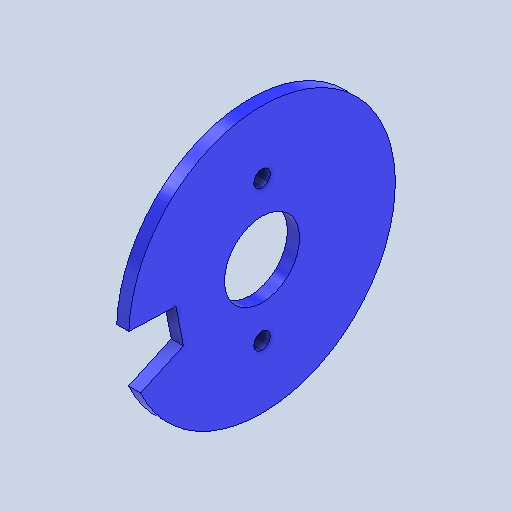
# Autodesk Inventor part: belt_liner_v2_3DP_P-2-F
Saved by Autodesk Inventor 2025.2 (Build 292293000, 293)
## iProperties
Created: 2025-01-13
Part Number: belt_liner_v2_3DP_P-2-F
Material: ABS プラスチック
Document SubType Name: Modeling
Designer: haruy
Density: 1.06 g/cm^3
Appearance: 青 - 壁塗料 - 光沢
Author: haruy
Autodesk Inventor part; units mm, degrees
ref_plane "YZ Plane" through (0, 0, 0) normal (1, 0, 0) x (0, 1, 0)
ref_plane "XZ Plane" through (0, 0, 0) normal (0, 1, 0) x (-1, 0, 0)
ref_plane "XY Plane" through (0, 0, 0) normal (0, 0, 1) x (1, 0, 0)
sketch "スケッチ1" plane through (0, 0, 0) normal (1, 0, 0) x (0, 1, 0)
  circle A0 centre (19.5992, 5.9415) radius 1.7
  circle A1 centre (-9.4008, 5.9415) radius 1.7
  line L0 (-2.2068, 22.1678) -> (-6.2315, 30.9988)
  arc A2 (-6.2315, 30.9988) -> (5.9783, 33.4275) centre (5.0992, 5.9415) ccw
  line L1 (5.6395, 23.7285) -> (-2.2068, 22.1678)
  circle A3 centre (5.0992, 5.9415) radius 7.75
  line L2 (5.9783, 33.4275) -> (5.6395, 23.7285)
  point P0 (0, 0)
  constraints: 6 end point, 4 centre point, 2 point on circle
extrude "押し出し1" add sketch "スケッチ1" along normal blind 2.5
